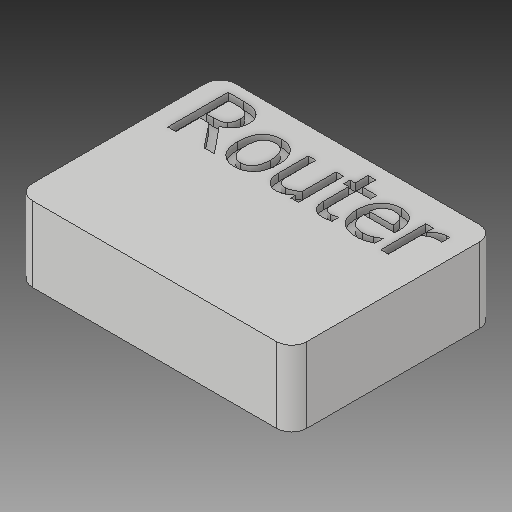
# Autodesk Inventor part: router-ver1-1111-2017
Saved by Autodesk Inventor 2017 (Build 210142000, 142)
## iProperties
Created: 2017-02-07
Part Number: router-ver1-1111-2017
Material: Generic
Document SubType Name: Modeling
Designer: 601898
Density: 1 g/cm^3
Appearance: Default
Author: 601898
Autodesk Inventor part; units mm, degrees
note: some values were not read from the file. Chosen so that the rebuilt part matches the saved one: direction of "Emboss1".
ref_plane "YZ Plane" through (0, 0, 0) normal (1, 0, 0) x (0, 1, 0)
ref_plane "XZ Plane" through (0, 0, 0) normal (0, 1, 0) x (-1, 0, 0)
ref_plane "XY Plane" through (0, 0, 0) normal (0, 0, 1) x (1, 0, 0)
sketch "Sketch1" plane through (0, 0, 0) normal (0, 1, 0) x (-1, 0, 0)
  line L0 (5.08, 0) -> (87.63, 0)
  line L1 (92.71, -5.08) -> (92.71, -63.5)
  line L2 (87.63, -68.58) -> (5.08, -68.58)
  line L3 (0, -63.5) -> (0, -5.08)
  arc A0 (92.71, -5.08) -> (87.63, 0) centre (87.63, -5.08) ccw
  arc A1 (87.63, -68.58) -> (92.71, -63.5) centre (87.63, -63.5) ccw
  arc A2 (5.08, 0) -> (0, -5.08) centre (5.08, -5.08) ccw
  arc A3 (0, -63.5) -> (5.08, -68.58) centre (5.08, -63.5) ccw
  point P0 (0, 0)
  point P1 (92.71, -68.58)
  point P2 (92.71, 0)
  point P3 (0, -68.58)
  dimension "d0" = 92.71
  dimension "d1" = 68.58
  dimension "d2" = 5.08
  constraints: 8 end point, 8 point on circle, 8 point on line, 8 tangent, 4 centre point, 3 equal radius, 2 parallel, 1 horizontal, 1 perpendicular
  measures "d0" distance of point (92.71, -68.58) point (0, -68.58)
  measures "d1" distance of point (92.71, 0) point (92.71, -68.58)
  measures "d2" radius of A0
extrude "Extrusion1" add sketch "Sketch1" along normal blind 25.4
sketch "Sketch2" plane through (0, 25.4, 0) normal (0, 1, 0) x (1, 0, 0)
  line L0 (-88.3931, 64.8083) -> (-14.3106, 64.8083) construction
  line L1 (-14.3106, 64.8083) -> (-14.3106, 10.6477) construction
  line L2 (-14.3106, 10.6477) -> (-88.3931, 10.6477) construction
  line L3 (-88.3931, 10.6477) -> (-88.3931, 64.8083) construction
  line L4 (-70.609, 44.4883) -> (-74.1164, 44.4883)
  line L5 (-74.1164, 44.4883) -> (-80.5384, 52.5735)
  line L6 (-80.5384, 52.5735) -> (-83.6342, 52.5735)
  line L7 (-83.6342, 52.5735) -> (-83.6342, 44.4883)
  line L8 (-83.6342, 44.4883) -> (-86.3347, 44.4883)
  line L9 (-86.3347, 44.4883) -> (-86.3347, 64.8083)
  line L10 (-86.3347, 64.8083) -> (-81.0983, 64.8083)
  spline S0 degree 2 poles (-81.0983, 64.8083) (-79.3528, 64.8083) (-76.9981, 64.4295) (-75.9277, 63.7379) knots 0 0 0 1 2 2 2
  spline S1 degree 2 poles (-75.9277, 63.7379) (-74.8574, 63.0463) (-73.6224, 60.8892) (-73.6224, 59.2919) knots 0 0 0 1 2 2 2
  spline S2 degree 2 poles (-73.6224, 59.2919) (-73.6224, 57.0689) (-75.8948, 54.0555) (-77.8379, 53.3309) knots 0 0 0 1 2 2 2
  line L11 (-77.8379, 53.3309) -> (-70.609, 44.4883)
  spline S3 degree 2 poles (-76.4382, 59.0778) (-76.4382, 59.9671) (-77.0639, 61.3338) (-77.7226, 61.7784) knots 0 0 0 1 2 2 2
  spline S4 degree 2 poles (-77.7226, 61.7784) (-78.299, 62.1571) (-79.8304, 62.47) (-80.9501, 62.47) knots 0 0 0 1 2 2 2
  line L12 (-80.9501, 62.47) -> (-83.6342, 62.47)
  line L13 (-83.6342, 62.47) -> (-83.6342, 54.8294)
  line L14 (-83.6342, 54.8294) -> (-81.263, 54.8294)
  spline S5 degree 2 poles (-81.263, 54.8294) (-80.0938, 54.8294) (-78.2331, 55.2411) (-77.5909, 55.8833) knots 0 0 0 1 2 2 2
  spline S6 degree 2 poles (-77.5909, 55.8833) (-76.9981, 56.4432) (-76.4382, 58.024) (-76.4382, 59.0778) knots 0 0 0 1 2 2 2
  spline S7 degree 2 poles (-56.6616, 52.1124) (-56.6616, 48.2592) (-60.3666, 44.0601) (-63.4624, 44.0601) knots 0 0 0 1 2 2 2
  spline S8 degree 2 poles (-63.4624, 44.0601) (-66.6405, 44.0601) (-70.2796, 48.3909) (-70.2796, 52.1124) knots 0 0 0 1 2 2 2
  spline S9 degree 2 poles (-70.2796, 52.1124) (-70.2796, 55.9327) (-66.5252, 60.1647) (-63.4624, 60.1647) knots 0 0 0 1 2 2 2
  spline S10 degree 2 poles (-63.4624, 60.1647) (-60.3666, 60.1647) (-56.6616, 55.9492) (-56.6616, 52.1124) knots 0 0 0 1 2 2 2
  spline S11 degree 2 poles (-59.3128, 52.1124) (-59.3128, 55.0764) (-61.4699, 57.9581) (-63.4624, 57.9581) knots 0 0 0 1 2 2 2
  spline S12 degree 2 poles (-63.4624, 57.9581) (-65.4549, 57.9581) (-67.6285, 55.0764) (-67.6285, 52.1124) knots 0 0 0 1 2 2 2
  spline S13 degree 2 poles (-67.6285, 52.1124) (-67.6285, 49.2307) (-65.4549, 46.2667) (-63.4624, 46.2667) knots 0 0 0 1 2 2 2
  spline S14 degree 2 poles (-63.4624, 46.2667) (-61.4864, 46.2667) (-59.3128, 49.1813) (-59.3128, 52.1124) knots 0 0 0 1 2 2 2
  line L15 (-42.1708, 44.4883) -> (-44.7397, 44.4883)
  line L16 (-44.7397, 44.4883) -> (-44.7397, 46.1679)
  spline S15 degree 2 poles (-44.7397, 46.1679) (-45.9253, 45.1305) (-48.0495, 44.0601) (-49.3668, 44.0601) knots 0 0 0 1 2 2 2
  spline S16 degree 2 poles (-49.3668, 44.0601) (-50.3548, 44.0601) (-52.1168, 44.7188) (-52.759, 45.4269) knots 0 0 0 1 2 2 2
  spline S17 degree 2 poles (-52.759, 45.4269) (-53.4177, 46.135) (-54.1422, 48.2921) (-54.1422, 49.84) knots 0 0 0 1 2 2 2
  line L17 (-54.1422, 49.84) -> (-54.1422, 59.7365)
  line L18 (-54.1422, 59.7365) -> (-51.5734, 59.7365)
  line L19 (-51.5734, 59.7365) -> (-51.5734, 51.0421)
  spline S18 degree 2 poles (-51.5734, 51.0421) (-51.5734, 49.8235) (-51.3922, 48.2262) (-51.0794, 47.6334) knots 0 0 0 1 2 2 2
  spline S19 degree 2 poles (-51.0794, 47.6334) (-50.7665, 47.0406) (-49.6962, 46.4972) (-48.6917, 46.4972) knots 0 0 0 1 2 2 2
  spline S20 degree 2 poles (-48.6917, 46.4972) (-47.7531, 46.4972) (-45.6289, 47.5676) (-44.7397, 48.3415) knots 0 0 0 1 2 2 2
  line L20 (-44.7397, 48.3415) -> (-44.7397, 59.7365)
  line L21 (-44.7397, 59.7365) -> (-42.1708, 59.7365)
  line L22 (-42.1708, 59.7365) -> (-42.1708, 44.4883)
  spline S21 degree 2 poles (-33.8387, 44.1919) (-35.9299, 44.1919) (-38.2847, 46.5796) (-38.2847, 49.1648) knots 0 0 0 1 2 2 2
  line L23 (-38.2847, 49.1648) -> (-38.2847, 57.6123)
  line L24 (-38.2847, 57.6123) -> (-40.0137, 57.6123)
  line L25 (-40.0137, 57.6123) -> (-40.0137, 59.7365)
  line L26 (-40.0137, 59.7365) -> (-38.2847, 59.7365)
  line L27 (-38.2847, 59.7365) -> (-38.2847, 64.1167)
  line L28 (-38.2847, 64.1167) -> (-35.7159, 64.1167)
  line L29 (-35.7159, 64.1167) -> (-35.7159, 59.7365)
  line L30 (-35.7159, 59.7365) -> (-30.9899, 59.7365)
  line L31 (-30.9899, 59.7365) -> (-30.9899, 57.6123)
  line L32 (-30.9899, 57.6123) -> (-35.7159, 57.6123)
  line L33 (-35.7159, 57.6123) -> (-35.7159, 50.3505)
  spline S22 degree 2 poles (-35.7159, 50.3505) (-35.7159, 49.1978) (-35.6335, 47.9298) (-35.3536, 47.3864) knots 0 0 0 1 2 2 2
  spline S23 degree 2 poles (-35.3536, 47.3864) (-35.1231, 46.9089) (-34.0857, 46.4314) (-33.1965, 46.4314) knots 0 0 0 1 2 2 2
  spline S24 degree 2 poles (-33.1965, 46.4314) (-32.5707, 46.4314) (-31.4016, 46.8101) (-31.1381, 46.9254) knots 0 0 0 1 2 2 2
  line L34 (-31.1381, 46.9254) -> (-30.9899, 46.9254)
  line L35 (-30.9899, 46.9254) -> (-30.9899, 44.62)
  spline S25 degree 2 poles (-30.9899, 44.62) (-31.7144, 44.4224) (-33.1965, 44.1919) (-33.8387, 44.1919) knots 0 0 0 1 2 2 2
  spline S26 degree 2 poles (-22.4766, 44.1425) (-26.1322, 44.1425) (-30.1501, 48.2427) (-30.1501, 52.0301) knots 0 0 0 1 2 2 2
  spline S27 degree 2 poles (-30.1501, 52.0301) (-30.1501, 55.7516) (-26.2475, 60.1647) (-23.1023, 60.1647) knots 0 0 0 1 2 2 2
  spline S28 degree 2 poles (-23.1023, 60.1647) (-21.6862, 60.1647) (-19.4961, 59.3413) (-18.6892, 58.4686) knots 0 0 0 1 2 2 2
  spline S29 degree 2 poles (-18.6892, 58.4686) (-17.8659, 57.5958) (-16.9931, 55.0764) (-16.9931, 53.2486) knots 0 0 0 1 2 2 2
  line L36 (-16.9931, 53.2486) -> (-16.9931, 51.8489)
  line L37 (-16.9931, 51.8489) -> (-27.5484, 51.8489)
  spline S30 degree 2 poles (-27.5484, 51.8489) (-27.5484, 49.1978) (-24.8807, 46.382) (-22.5095, 46.382) knots 0 0 0 1 2 2 2
  spline S31 degree 2 poles (-22.5095, 46.382) (-21.6697, 46.382) (-20.0395, 46.7607) (-19.3808, 47.0571) knots 0 0 0 1 2 2 2
  spline S32 degree 2 poles (-19.3808, 47.0571) (-18.6892, 47.3864) (-17.7342, 47.9628) (-17.4213, 48.2262) knots 0 0 0 1 2 2 2
  line L38 (-17.4213, 48.2262) -> (-17.2731, 48.2262)
  line L39 (-17.2731, 48.2262) -> (-17.2731, 45.4269)
  spline S33 degree 2 poles (-17.2731, 45.4269) (-17.7177, 45.2458) (-19.068, 44.7188) (-19.5949, 44.5706) knots 0 0 0 1 2 2 2
  spline S34 degree 2 poles (-19.5949, 44.5706) (-20.3359, 44.3565) (-21.5544, 44.1425) (-22.4766, 44.1425) knots 0 0 0 1 2 2 2
  spline S35 degree 2 poles (-19.4961, 53.8085) (-19.529, 54.8459) (-19.9572, 56.3608) (-20.3688, 56.8713) knots 0 0 0 1 2 2 2
  spline S36 degree 2 poles (-20.3688, 56.8713) (-20.8134, 57.4476) (-22.2131, 58.0569) (-23.2505, 58.0569) knots 0 0 0 1 2 2 2
  spline S37 degree 2 poles (-23.2505, 58.0569) (-24.2715, 58.0569) (-25.7041, 57.4476) (-26.2969, 56.8548) knots 0 0 0 1 2 2 2
  spline S38 degree 2 poles (-26.2969, 56.8548) (-26.8732, 56.2456) (-27.466, 54.78) (-27.5484, 53.8085) knots 0 0 0 1 2 2 2
  line L40 (-27.5484, 53.8085) -> (-19.4961, 53.8085)
  line L41 (-6.3062, 56.9866) -> (-6.4379, 56.9866)
  spline S39 degree 2 poles (-6.4379, 56.9866) (-6.7343, 57.0689) (-7.3766, 57.1018) (-7.8212, 57.1018) knots 0 0 0 1 2 2 2
  spline S40 degree 2 poles (-7.8212, 57.1018) (-8.8586, 57.1018) (-10.9004, 56.1962) (-11.8226, 55.307) knots 0 0 0 1 2 2 2
  line L42 (-11.8226, 55.307) -> (-11.8226, 44.4883)
  line L43 (-11.8226, 44.4883) -> (-14.3914, 44.4883)
  line L44 (-14.3914, 44.4883) -> (-14.3914, 59.7365)
  line L45 (-14.3914, 59.7365) -> (-11.8226, 59.7365)
  line L46 (-11.8226, 59.7365) -> (-11.8226, 57.4641)
  spline S41 degree 2 poles (-11.8226, 57.4641) (-10.4229, 58.7156) (-8.3316, 59.7365) (-7.3436, 59.7365) knots 0 0 0 1 2 2 2
  spline S42 degree 2 poles (-7.3436, 59.7365) (-6.9484, 59.7365) (-6.5532, 59.7036) (-6.3062, 59.6542) knots 0 0 0 1 2 2 2
  line L47 (-6.3062, 59.6542) -> (-6.3062, 56.9866)
  point P0 (0, 0)
  constraints: 2 other
emboss "Emboss1" sketch "Sketch2" operation cut depth 2.54 direction (0, -1, 0)
body "Solid1"
